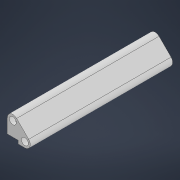
# Autodesk Inventor part: radiator_adapter_01
Saved by Autodesk Inventor 2022 (Build 260153000, 153)
## iProperties
Created: 2025-02-03
Part Number: radiator_adapter_01
Material: 一般
Document SubType Name: Modeling
Designer: gisen
Density: 1 g/cm^3
Appearance: 既定
Author: gisen
Autodesk Inventor part; units mm, degrees
ref_plane "YZ Plane" through (0, 0, 0) normal (1, 0, 0) x (0, 1, 0)
ref_plane "XZ Plane" through (0, 0, 0) normal (0, 1, 0) x (-1, 0, 0)
ref_plane "XY Plane" through (0, 0, 0) normal (0, 0, 1) x (1, 0, 0)
sketch "スケッチ1" plane through (0, 0, 0) normal (0, 0, 1) x (1, 0, 0)
  circle A0 centre (250, -200) radius 1.6 construction
  circle A1 centre (239, -189) radius 1.6 construction
  circle A2 centre (250, -200) radius 3.2
  circle A3 centre (239, -189) radius 3.2
  circle A4 centre (250, -200) radius 5 construction
  circle A5 centre (239, -189) radius 5 construction
  line L0 (242.5355, -185.4645) -> (253.5355, -196.4645)
  line L1 (250, -200) -> (239, -189) construction
  line L2 (-250, -205) -> (250, -205) projected
  line L3 (244, -202) -> (234, -202)
  line L4 (234, -202) -> (234, -189)
  line L5 (244, -202) -> (244, -205)
  line L6 (244, -205) -> (250, -205)
  arc A6 (250, -205) -> (253.5355, -196.4645) centre (250, -200) ccw
  arc A7 (242.5355, -185.4645) -> (234, -189) centre (239, -189) ccw
  point P0 (0, 0)
  point P1 (255, -200)
  dimension "d0" = 6.4
  dimension "d2" = 10
  dimension "d3" = 3
  constraints: 12 end point, 8 point on circle, 6 centre point, 6 coincident, 4 tangent, 2 equal radius, 1 collinear, 1 perpendicular, 1 point on line, 1 vertical, 1 other
  measures "d0" diameter of A2
  measures "d2" distance between parallel lines of L4 L5
  measures "d3" distance of L3.start L5.end
extrude "押し出し1" add sketch "スケッチ1" along normal blind 130
sketch "スケッチ2" plane through (234, -202, 0) normal (0, -1, 0) x (1, 0, 0)
  line L0 (1.8, 130) -> (8.2, 130) construction
  line L1 (1.8, 0) -> (8.2, 0) construction
  line L2 (5, 130) -> (5, 0) construction
  circle A0 centre (5, 125) radius 2.25
  circle A1 centre (5, 5) radius 2.25
  point P0 (-234, 0)
  dimension "d6" = 4.5
  dimension "d7" = 5
  dimension "d8" = 5
  constraints: 2 centre point, 2 end point, 2 midpoint, 2 point on line, 1 equal radius
  measures "d6" diameter of A0
  measures "d7" distance from line of A0.centre L0
  measures "d8" distance of L2.end A1.centre
extrude "押し出し2" cut sketch "スケッチ2" against normal blind 5
sketch "スケッチ3" plane through (234, -202, 0) normal (0, -1, 0) x (1, 0, 0)
  circle A0 centre (5, 125) radius 2.25 construction
  circle A1 centre (5, 5) radius 2.25 construction
  circle A2 centre (5, 125) radius 1.6
  circle A3 centre (5, 5) radius 1.6
  point P0 (-234, 0)
  dimension "d11" = 3.2
  constraints: 2 centre point, 2 coincident, 1 equal radius
  measures "d11" diameter of A2
extrude "押し出し3" cut sketch "スケッチ3" against normal blind 13
equation "\"d8\" = d7"
